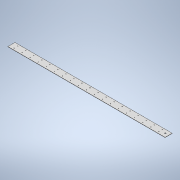
# Autodesk Inventor part: Assembly_plate_beamV3
Saved by Autodesk Inventor 2022 (Build 260153000, 153)
## iProperties
Created: 2022-04-25
Part Number: Assembly_plate_beamV3
Material: Generic
Document SubType Name: Sheet Metal
Designer: Patrick
Density: 1 g/cm^3
Sheet Metal Rule: Default_mm
Appearance: Default
Author: Patrick
Autodesk Inventor part; units mm, degrees
ref_plane "YZ Plane" through (0, 0, 0) normal (1, 0, 0) x (0, 1, 0)
ref_plane "XZ Plane" through (0, 0, 0) normal (0, 1, 0) x (-1, 0, 0)
ref_plane "XY Plane" through (0, 0, 0) normal (0, 0, 1) x (1, 0, 0)
sketch "Sketch1" plane through (0, 0, 0) normal (0, 1, 0) x (-1, 0, 0)
  line L0 (0, 0) -> (978, 0)
  line L1 (978, 0) -> (978, -44)
  line L2 (978, -44) -> (0, -44)
  line L3 (0, -44) -> (0, 0)
  circle A0 centre (950, -11) radius 1.675
  circle A1 centre (900, -11) radius 1.675
  circle A2 centre (850, -11) radius 1.675
  circle A3 centre (800, -11) radius 1.675
  circle A4 centre (750, -11) radius 1.675
  circle A5 centre (700, -11) radius 1.675
  circle A6 centre (650, -11) radius 1.675
  circle A7 centre (600, -11) radius 1.675
  circle A8 centre (550, -11) radius 1.675
  circle A9 centre (500, -11) radius 1.675
  circle A10 centre (450, -11) radius 1.675
  circle A11 centre (400, -11) radius 1.675
  circle A12 centre (350, -11) radius 1.675
  circle A13 centre (300, -11) radius 1.675
  circle A14 centre (250, -11) radius 1.675
  circle A15 centre (200, -11) radius 1.675
  circle A16 centre (150, -11) radius 1.675
  circle A17 centre (100, -11) radius 1.675
  circle A18 centre (50, -11) radius 1.675
  circle A19 centre (950, -33) radius 1.675
  circle A20 centre (900, -33) radius 1.675
  circle A21 centre (850, -33) radius 1.675
  circle A22 centre (800, -33) radius 1.675
  circle A23 centre (750, -33) radius 1.675
  circle A24 centre (700, -33) radius 1.675
  circle A25 centre (650, -33) radius 1.675
  circle A26 centre (600, -33) radius 1.675
  circle A27 centre (550, -33) radius 1.675
  circle A28 centre (500, -33) radius 1.675
  circle A29 centre (450, -33) radius 1.675
  circle A30 centre (400, -33) radius 1.675
  circle A31 centre (350, -33) radius 1.675
  circle A32 centre (300, -33) radius 1.675
  circle A33 centre (250, -33) radius 1.675
  circle A34 centre (200, -33) radius 1.675
  circle A35 centre (150, -33) radius 1.675
  circle A36 centre (100, -33) radius 1.675
  circle A37 centre (50, -33) radius 1.675
  circle A38 centre (20, -22) radius 4
  dimension "d0" = 44
  dimension "d1" = 978
  dimension "d2" = 11
  dimension "d3" = 28
  dimension "d4" = 3.35
  dimension "d7" = 50
  dimension "d10" = 22
  dimension "d16" = 8
  dimension "d17" = 20
  dimension "d18" = 22
  measures "d0" distance of L2.end L0.start
  measures "d1" distance of L1.end L2.end
  measures "d2" distance from line of L0 A0.centre
  measures "d3" distance from line of L1 A0.centre
  measures "d4" diameter of A0
  measures "d7" distance of A0.centre A1.centre
  measures "d10" distance of A0.centre A19.centre
  measures "d16" diameter of A38
  measures "d17" distance from line of A38.centre L3
  measures "d18" distance from line of A38.centre L2
extrude "Plate4" add sketch "Sketch1" along normal blind 1.5
equation "\"d18\" = 0.5 * d0"
equation "\"d19\" = Thickness"
equation "\"BendRadius\" = Thickness"
equation "\"BendReliefWidth\" = Thickness"
equation "\"BendReliefDepth\" = 0.5 * Thickness"
equation "\"CornerReliefSize\" = 4 * Thickness"
equation "\"MinimumRemnant\" = 2 * Thickness"
equation "\"TransitionRadius\" = BendRadius"
equation "\"JacobiRadiusSize\" = BendRadius"
equation "\"GapSize\" = Thickness"
equation "\"Thickness\" = 1.5"
body "Solid4"
